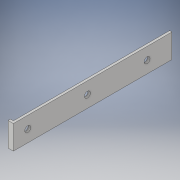
# Autodesk Inventor part: Chapa da Caixa de Segurança
Saved by Autodesk Inventor 2019 (Build 230136000, 136)
## iProperties
Created: 2020-06-15
Part Number: Chapa da Caixa de Segurança
Material: Genérico
Document SubType Name: Modeling
Designer: lukas
Density: 1 g/cm^3
Appearance: Padrão
Author: lukas
Autodesk Inventor part; units mm, degrees
ref_plane "YZ Plane" through (0, 0, 0) normal (1, 0, 0) x (0, 1, 0)
ref_plane "XZ Plane" through (0, 0, 0) normal (0, 1, 0) x (-1, 0, 0)
ref_plane "XY Plane" through (0, 0, 0) normal (0, 0, 1) x (1, 0, 0)
sketch "Esboço1" plane through (0, 0, 0) normal (1, 0, 0) x (0, 1, 0)
  line L0 (0, 0) -> (20, 0)
  line L1 (20, 0) -> (20, -132.9)
  line L2 (20, -132.9) -> (0, -132.9)
  line L3 (0, -132.9) -> (0, 0)
  line L4 (10, -132.9) -> (10, -62)
  circle A0 centre (10, -62) radius 2.5
  line L5 (10, -62) -> (10, -12)
  circle A1 centre (10, -12) radius 2.5
  dimension "d0" = 20
  dimension "d1" = 132.9
  dimension "d2" = 70.9
  dimension "d3" = 5
  dimension "d4" = 50
  dimension "d5" = 5
  constraints: 12 end point, 2 centre point, 2 coincident, 2 parallel, 2 vertical, 1 horizontal, 1 midpoint, 1 perpendicular
  measures "d0" distance of L1.end L2.end
  measures "d1" distance of L0.end L1.end
  measures "d2" distance of L4.start L4.end
  measures "d3" diameter of A0
  measures "d4" distance of L5.start L5.end
  measures "d5" diameter of A1
extrude "Extrusão1" add sketch "Esboço1" along normal blind 2
sketch "Esboço2" plane through (0, 0, 0) normal (0, 0, 1) x (1, 0, 0)
  line L0 (2, 20) -> (2, 0) projected
  line L1 (2, 0) -> (-2.5, 0)
  line L2 (-2.5, 0) -> (-2.5, 20)
  line L3 (-2.5, 20) -> (2, 20)
  line L4 (2, 20) -> (2, 0)
  point P0 (0, 0)
  dimension "d8" = 4.5
  constraints: 8 end point, 2 parallel, 1 horizontal, 1 perpendicular
  measures "d8" distance of L2.end L3.end
extrude "Extrusão2" add sketch "Esboço2" against normal blind 2
sketch "Esboço3" plane through (2, 0, 0) normal (1, 0, 0) x (0, 0, -1)
  circle A0 centre (12, 10) radius 2.5 projected
  circle A1 centre (12, 10) radius 2.5
  circle A2 centre (62, 10) radius 2.5 projected
  circle A3 centre (62, 10) radius 2.5
  line L0 (62, 10) -> (112, 10) construction
  point P0 (0, 0)
  dimension "d11" = 50
  constraints: 2 centre point, 2 coincident, 2 end point, 1 horizontal
  measures "d11" distance of L0.start L0.end
hole "Furo1" at (2, 10, -112) direction (-1, 0, 0) diameter 5 end through all
